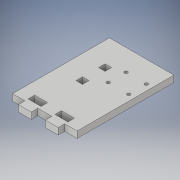
# Autodesk Inventor part: thumper-bumper-sidewall-v2
Saved by Autodesk Inventor 2017 (Build 210142000, 142)
## iProperties
Created: 2017-02-22
Part Number: thumper-bumper-sidewall-v2
Material: Generic
Document SubType Name: Modeling
Designer: John
Density: 1 g/cm^3
Appearance: Default
Author: John
Autodesk Inventor part; units mm, degrees
ref_plane "YZ Plane" through (0, 0, 0) normal (1, 0, 0) x (0, 1, 0)
ref_plane "XZ Plane" through (0, 0, 0) normal (0, 1, 0) x (-1, 0, 0)
ref_plane "XY Plane" through (0, 0, 0) normal (0, 0, 1) x (1, 0, 0)
sketch "Sketch1" plane through (0, 0, 0) normal (0, 1, 0) x (-1, 0, 0)
  line L0 (27.5, -0.0615) -> (27.5, 89.9385)
  line L1 (-32.5, 89.9385) -> (-32.5, -0.0615)
  line L2 (-32.5, -0.0615) -> (-2.5, -0.0615)
  line L3 (-2.5, -0.0615) -> (-2.5, 89.9385) construction
  line L4 (-32.5, 44.9385) -> (-2.5, 44.9385) construction
  line L5 (-32.5, 89.9385) -> (27.5, 89.9385)
  line L6 (-21, 89.9385) -> (-9, 89.9385)
  line L7 (-9, 89.9385) -> (-9, 95.9385)
  line L8 (-9, 95.9385) -> (-21, 95.9385)
  line L9 (-21, 95.9385) -> (-21, 89.9385)
  line L10 (16, 89.9385) -> (4, 89.9385)
  line L11 (4, 89.9385) -> (4, 95.9385)
  line L12 (4, 95.9385) -> (16, 95.9385)
  line L13 (16, 95.9385) -> (16, 89.9385)
  line L14 (-2.5, 44.9385) -> (27.5, 44.9385) construction
  line L15 (-2.5, -0.0615) -> (27.5, -0.0615)
  line L16 (-9, 86.9385) -> (-21, 86.9385)
  line L17 (-21, 86.9385) -> (-21, 80.9385)
  line L18 (-21, 80.9385) -> (-9, 80.9385)
  line L19 (-9, 80.9385) -> (-9, 86.9385)
  line L20 (-9, 86.9385) -> (-21, 80.9385) construction
  line L21 (-21, 86.9385) -> (-9, 80.9385) construction
  line L22 (4, 86.9385) -> (16, 86.9385)
  line L23 (16, 86.9385) -> (16, 80.9385)
  line L24 (16, 80.9385) -> (4, 80.9385)
  line L25 (4, 80.9385) -> (4, 86.9385)
  line L26 (4, 86.9385) -> (16, 80.9385) construction
  line L27 (16, 86.9385) -> (4, 80.9385) construction
  point P0 (-15, 83.9385)
  point P1 (10, 83.9385)
  dimension "d0" = 60
  dimension "d1" = 90
  dimension "d18" = 12
  dimension "d19" = 6
  dimension "d20" = 18.5
  dimension "d21" = 12
  dimension "d22" = 6
  dimension "d23" = 3
  constraints: 56 end point, 9 symmetric about line, 7 midpoint, 7 parallel, 5 horizontal, 2 equal length, 2 perpendicular, 1 collinear, 1 point on line, 1 vertical
  measures "d0" distance of L1.start L0.end
  measures "d1" distance of L0.end L0.start
  measures "d18" distance of L8.end L7.end
  measures "d19" distance of L7.end L6.end
  measures "d20" distance between parallel lines of L3 L9
  measures "d21" distance of L18.end L17.end
  measures "d22" distance of L17.end L16.end
  measures "d23" distance between parallel lines of L5 L16
extrude "Extrusion1" add sketch "Sketch1" along normal blind 6
sketch "Sketch2" plane through (0, 6, 0) normal (0, 1, 0) x (1, 0, 0)
  circle A0 centre (8, -19.9385) radius 1.4986
  circle A1 centre (27, -19.9385) radius 1.4986
  circle A2 centre (27, -36.4385) radius 1.4985
  circle A3 centre (8, -36.4385) radius 1.4985
  line L0 (27, -36.4385) -> (8, -36.4385) construction
  line L1 (8, -36.4385) -> (8, -19.9385) construction
  line L2 (8, -19.9385) -> (27, -19.9385) construction
  line L3 (27, -19.9385) -> (27, -36.4385) construction
  line L4 (27, -36.4385) -> (8, -19.9385) construction
  line L5 (27, -19.9385) -> (8, -36.4385) construction
  line L6 (32.5, 0.0615) -> (-27.5, 0.0615) construction
  line L7 (2.5, 0.0615) -> (2.5, -89.9385) construction
  line L8 (-4, -89.9385) -> (9, -89.9385) construction
  line L9 (-2.5, -49.9385) -> (-8.5, -49.9385)
  line L10 (-8.5, -49.9385) -> (-8.5, -43.9385)
  line L11 (-8.5, -43.9385) -> (-2.5, -43.9385)
  line L12 (-2.5, -43.9385) -> (-2.5, -49.9385)
  line L13 (-2.5, -28.9385) -> (-8.5, -28.9385)
  line L14 (-8.5, -28.9385) -> (-8.5, -22.9385)
  line L15 (-8.5, -22.9385) -> (-2.5, -22.9385)
  line L16 (-2.5, -22.9385) -> (-2.5, -28.9385)
  point P0 (0, 0)
  point P1 (17.5, -28.1885)
  dimension "d26" = 2.9972
  dimension "d28" = 2.9972
  dimension "d29" = 19
  dimension "d30" = 2.997
  dimension "d31" = 2.997
  dimension "d32" = 16.5
  dimension "d33" = 15
  dimension "d36" = 20
  dimension "d37" = 6
  dimension "d38" = 6
  dimension "d39" = 6
  dimension "d40" = 5
  dimension "d41" = 40
  dimension "d42" = 15
  constraints: 30 end point, 5 perpendicular, 4 centre point, 4 parallel, 3 horizontal, 3 midpoint, 2 point on line
  measures "d26" diameter of A0
  measures "d28" diameter of A1
  measures "d29" distance of L1.end L2.end
  measures "d30" diameter of A3
  measures "d31" diameter of A2
  measures "d32" distance of L2.end L0.start
  measures "d33" distance from line of L7 point (17.5, -28.189)
  measures "d36" distance between parallel lines of L6 L2
  measures "d37" distance of L10.end L11.end
  measures "d38" distance of L9.end L10.end
  measures "d39" distance of L13.end L14.end
  measures "d40" distance between parallel lines of L7 L12
  measures "d41" distance between parallel lines of L8 L9
  measures "d42" distance between parallel lines of L11 L13
extrude "Extrusion2" cut sketch "Sketch2" against normal through all
body "Solid1"
